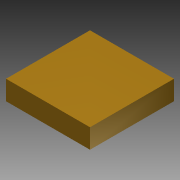
# Autodesk Inventor part: DemoSimpleSurfaceGraphics
Saved by Autodesk Inventor 2012 (Build 160160000, 160)
## iProperties
Created: 2011-09-20
Part Number: DemoSimpleSurfaceGraphics
Material: Default
Document SubType Name: Modeling
Designer: Felipe
Density: 1 g/cm^3
Author: Felipe
Autodesk Inventor part; units mm, degrees
ref_plane "YZ Plane" through (0, 0, 0) normal (1, 0, 0) x (0, 1, 0)
ref_plane "XZ Plane" through (0, 0, 0) normal (0, 1, 0) x (-1, 0, 0)
ref_plane "XY Plane" through (0, 0, 0) normal (0, 0, 1) x (1, 0, 0)
sketch "Sketch1" plane through (0, 0, 0) normal (0, 0, 1) x (1, 0, 0)
  line L0 (-27.094, 22.2533) -> (16.108, 22.2533)
  line L1 (16.108, 22.2533) -> (16.108, -20.9488)
  line L2 (16.108, -20.9488) -> (-27.094, -20.9488)
  line L3 (-27.094, -20.9488) -> (-27.094, 22.2533)
  point P0 (0, 0)
  constraints: 8 end point, 2 parallel, 2 perpendicular, 1 horizontal
extrude "Extrusion1" add sketch "Sketch1" along normal blind 10
body "Solid1"
